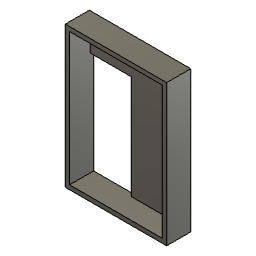
PCB_Case v1 (Autodesk Fusion 360 design; units mm, degrees)
Autodesk Fusion 360 part; units mm, degrees
other "Base Mesh Feature1"
other "Modify1"
other "Modify2"
other "Modify3"
other "Modify4"
sketch "Sketch1" plane through (0, 0, 0) normal (0, 0, 1) x (1, 0, 0)
  line L0 (50.6093, 116.6151) -> (104.5154, 116.6151)
  line L1 (104.5154, 116.6151) -> (104.5154, 39.506)
  line L2 (104.5154, 39.506) -> (50.6093, 39.506)
  line L3 (50.6093, 39.506) -> (50.6093, 116.6151)
  line L4 (48.1093, 119.1151) -> (107.0154, 119.1151)
  line L5 (107.0154, 119.1151) -> (107.0154, 37.006)
  line L6 (107.0154, 37.006) -> (48.1093, 37.006)
  line L7 (48.1093, 37.006) -> (48.1093, 119.1151)
  dimension "d1" = 2.5
  dimension "d2" = 2.5
  dimension "d3" = 2.5
  dimension "d4" = 2.5
  constraint horizontal L0
  constraint vertical L1
  constraint horizontal L2
  constraint vertical L3
  constraint horizontal L4
  constraint vertical L5
  constraint horizontal L6
  constraint vertical L7
  measures "d1" distance of L0 L4
  measures "d2" distance of L3 L7
  measures "d3" distance of L2 L6
  measures "d4" distance of L1 L5
extrude "Extrude1" add sketch "Sketch1" along normal blind 12
sketch "Sketch2" plane through (0, 0, 0) normal (0, 0, -1) x (-1, 0, 0)
  line L0 (-50.6093, 39.506) -> (-104.5154, 39.506)
  line L1 (-104.5154, 39.506) -> (-104.5154, 116.6151)
  line L2 (-104.5154, 116.6151) -> (-50.6093, 116.6151)
  line L3 (-50.6093, 116.6151) -> (-50.6093, 39.506)
  line L4 (-107.0154, 37.006) -> (-48.1093, 37.006)
  line L5 (-48.1093, 37.006) -> (-48.1093, 119.1151)
  line L6 (-48.1093, 119.1151) -> (-107.0154, 119.1151)
  line L7 (-107.0154, 119.1151) -> (-107.0154, 37.006)
  line L8 (-48.1093, 37.006) -> (-107.0154, 37.006)
  line L9 (-107.0154, 37.006) -> (-107.0154, 119.1151)
  line L10 (-107.0154, 119.1151) -> (-48.1093, 119.1151)
  line L11 (-48.1093, 119.1151) -> (-48.1093, 37.006)
  line L12 (-50.6093, 39.506) -> (-74.4442, 39.506)
  line L13 (-74.4442, 39.506) -> (-74.4442, 99.7953)
  line L14 (-74.4442, 99.7953) -> (-50.6093, 99.7953)
  line L15 (-50.6093, 99.7953) -> (-50.6093, 39.506)
  constraint horizontal L8
  constraint vertical L9
  constraint horizontal L10
  constraint vertical L11
  constraint coincident L6.end L7.start
  constraint coincident L4.end L5.start
  constraint horizontal L12
  constraint vertical L13
  constraint horizontal L14
  constraint vertical L15
  constraint coincident L0.start L3.end
extrude "Extrude2" add sketch "Sketch2" along normal blind 2 contours L0 L1 L2 L3 L13 L14 | L4 L5 L6 L7 L8 L9 L10 L11
